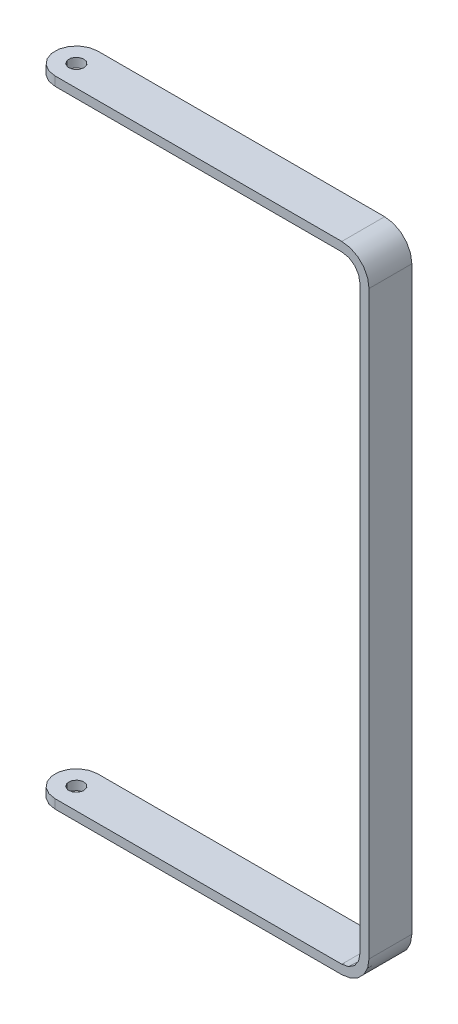
# Autodesk Inventor part: Pivoting Bracket
Saved by Autodesk Inventor 2024 (Build 280153000, 153)
## iProperties
Created: 2024-08-21
Part Number: Pivoting Bracket
Material: Generic
Document SubType Name: Modeling
Designer: Stefano
Density: 1 g/cm^3
Appearance: Default
Author: Stefano
Autodesk Inventor part; units mm, degrees
ref_plane "YZ Plane" through (0, 0, 0) normal (1, 0, 0) x (0, 1, 0)
ref_plane "XZ Plane" through (0, 0, 0) normal (0, 1, 0) x (-1, 0, 0)
ref_plane "XY Plane" through (0, 0, 0) normal (0, 0, 1) x (1, 0, 0)
ref_plane "Work Plane1" through (122.7733, 133.3708, 9.0922) normal (0, 0, 1) x (1, 0, 0)
sketch "Sketch1" plane through (122.7733, 133.3708, 9.0922) normal (0, 0, 1) x (1, 0, 0)
  line L0 (-23.375, 1.75) -> (-8.375, 1.75) construction
  line L1 (-8.375, -214.25) -> (-23.375, -214.25) construction
  line L2 (-23.375, 1.75) -> (84.575, 1.75)
  line L3 (90.925, -4.6) -> (90.925, -207.9)
  line L4 (84.575, -214.25) -> (-23.375, -214.25)
  arc A0 (90.925, -4.6) -> (84.575, 1.75) centre (84.575, -4.6) ccw
  arc A1 (84.575, -214.25) -> (90.925, -207.9) centre (84.575, -207.9) ccw
  point P0 (-122.7733, -133.3708)
  point P1 (90.925, 1.75)
  point P2 (90.925, -214.25)
  dimension "d0" = 114.3
  dimension "d3" = 6.35
  constraints: 6 end point, 4 point on circle, 4 point on line, 4 tangent, 2 centre point, 1 collinear, 1 equal radius, 1 horizontal, 1 perpendicular
  measures "d0" distance of L0.start point (90.925, 1.75)
  measures "d3" radius of A0
ref_plane "Work Plane3" through (99.3983, 135.1208, 9.0922) normal (-1, 0, 0) x (0, 1, 0)
ref_plane "Work Plane2" through (44.8233, 115.6208, -3.6078) normal (-1, 0, 0) x (0, 1, 0)
sketch "Sketch3" plane through (99.3983, 135.1208, 9.0922) normal (-1, 0, 0) x (0, 1, 0)
  line L0 (3.175, -7.5) -> (0, -7.5)
  line L1 (0, -7.5) -> (0, 7.5)
  line L2 (0, 7.5) -> (3.175, 7.5)
  line L3 (3.175, 7.5) -> (3.175, -7.5)
  line L4 (0, 7.5) -> (0, -7.5) projected
  point P0 (-135.1208, 9.0922)
  dimension "d4" = 3.175
  constraints: 8 end point, 2 parallel, 2 point on line, 1 collinear, 1 horizontal, 1 perpendicular
  measures "d4" distance between parallel lines of L3 L1
sweep "Sweep1" add profiles "Sketch3" path "Sketch1" path curves L2 A0 L3 A1 L4
fillet "Fillet1" radius 7.5 4 edges at (99.3983, 136.7083, 1.5922) (99.3983, 136.7083, 16.5922) (99.3983, -82.4667, 1.5922) (99.3983, -82.4667, 16.5922)
sketch "Sketch4" plane through (207.3483, -84.0542, 1.5922) normal (0, -1, 0) x (1, 0, 0)
  circle A0 centre (-100.45, 7.5) radius 2.7559 projected
  point P0 (-207.3483, -1.5922)
hole "Hole1" at (106.8983, -84.0542, 9.0922) direction (0, 1, 0) diameter 5.3086 depth 3.175 tip angle 118
ref_plane "Work Plane4" through (207.3483, 27.1208, 16.5922) normal (0, 1, 0) x (1, 0, 0)
mirror "Mirror1" about plane through (207.3483, 27.1208, 16.5922) normal (0, 1, 0) of "Hole1"
body "Solid1"
